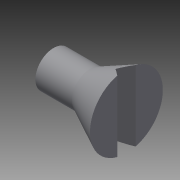
# Autodesk Inventor part: Hand
Saved by Autodesk Inventor 2015 (Build 190159000, 159)
## iProperties
Created: 2015-03-12
Part Number: Hand
Material: Generic
Document SubType Name: Modeling
Designer: pltwe4
Density: 1 g/cm^3
Appearance: Default
Author: pltwe4
Autodesk Inventor part; units mm, degrees
ref_plane "YZ Plane" through (0, 0, 0) normal (1, 0, 0) x (0, 1, 0)
ref_plane "XZ Plane" through (0, 0, 0) normal (0, 1, 0) x (-1, 0, 0)
ref_plane "XY Plane" through (0, 0, 0) normal (0, 0, 1) x (1, 0, 0)
sketch "Sketch1" plane through (0, 0, 0) normal (1, 0, 0) x (0, 1, 0)
  circle A0 centre (0, 0) radius 4
  circle A1 centre (0, 0) radius 5
  dimension "d0" = 8
  dimension "d1" = 10
  constraints: 2 centre point, 2 coincident
  measures "d0" diameter of A0
  measures "d1" diameter of A1
extrude "Extrusion1" add sketch "Sketch1" along normal blind 10
sketch "Sketch2" plane through (10, 0, 0) normal (1, 0, 0) x (0, 0, -1)
  circle A0 centre (0, 0) radius 4 projected
  circle A1 centre (0, 0) radius 5 projected
extrude "Extrusion2" add sketch "Sketch2" along normal blind 10 contours A0 | A1
sketch "Sketch3" plane through (20, 0, 0) normal (1, 0, 0) x (0, 0, -1)
  circle A0 centre (0, 0) radius 10
  dimension "d6" = 20
  constraints: 1 centre point, 1 coincident
  measures "d6" diameter of A0
loft "Loft1" add profiles "Sketch2", "Sketch3" contours A0 | A1 / all
sketch "Sketch4" plane through (0, 0, 0) normal (0, 0, 1) x (1, 0, 0)
  line L0 (10, 5) -> (10, -5) projected
  line L1 (20, 10) -> (20, -10) projected
  line L2 (-4, 0) -> (24, 0) projected
  line L3 (20, 2.5) -> (17, 0)
  line L4 (20, 10) -> (20, -10) projected
  line L5 (20, -2.5) -> (17, 0)
  line L6 (20, 2.5) -> (20, -2.5)
  point P0 (0, 0)
  dimension "d11" = 5
  dimension "d12" = 3
  constraints: 6 end point, 3 point on line, 1 collinear, 1 other
  measures "d11" distance of L5.start L3.start
  measures "d12" distance from line of L1 L3.end
extrude "Extrusion3" cut sketch "Sketch4" along normal mid plane 20
body "Solid1"
